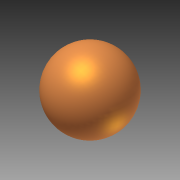
# Autodesk Inventor part: Compressed ball
Saved by Autodesk Inventor 2012 (Build 160160000, 160)
## iProperties
Created: 2012-01-10
Part Number: Compressed ball
Material: Default
Document SubType Name: Modeling
Designer: Justin
Density: 1 g/cm^3
Author: Justin
Autodesk Inventor part; units mm, degrees
ref_plane "YZ Plane" through (0, 0, 0) normal (1, 0, 0) x (0, 1, 0)
ref_plane "XZ Plane" through (0, 0, 0) normal (0, 1, 0) x (-1, 0, 0)
ref_plane "XY Plane" through (0, 0, 0) normal (0, 0, 1) x (1, 0, 0)
sketch "Sketch1" plane through (0, 0, 0) normal (0, 0, 1) x (1, 0, 0)
  arc A0 (0, 95.25) -> (0, -95.25) centre (0, 0) ccw
  line L0 (0, 95.25) -> (0, -95.25)
  dimension "d0" = 190.5
  dimension "d0" = 190.5
  constraints: 2 end point, 2 point on circle, 1 centre point, 1 coincident, 1 vertical
  measures "d0" diameter of A0
revolve "Revolution1" add sketch "Sketch1" angle 360 about axis through (0, 95.25, 0) along (0, -1, 0)
body "Solid1"
